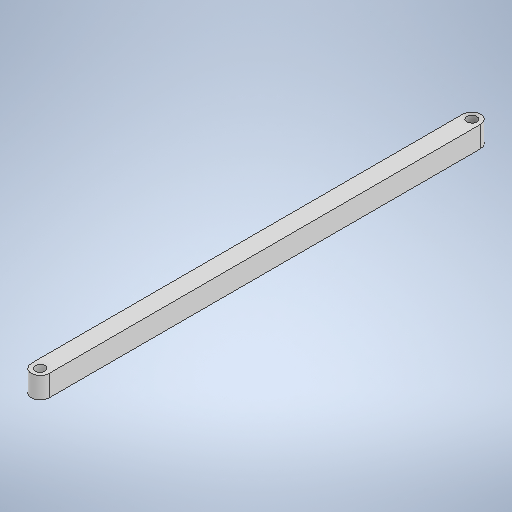
# Autodesk Inventor part: scrambler_spider_support1
Saved by Autodesk Inventor 2025.2 (Build 292293000, 293)
## iProperties
Created: 2025-10-14
Part Number: scrambler_spider_support1
Material: Generic
Document SubType Name: Modeling
Designer: pascu
Density: 1 g/cm^3
Appearance: Default
Author: pascu
Autodesk Inventor part; units mm, degrees
ref_plane "YZ Plane" through (0, 0, 0) normal (1, 0, 0) x (0, 1, 0)
ref_plane "XZ Plane" through (0, 0, 0) normal (0, 1, 0) x (-1, 0, 0)
ref_plane "XY Plane" through (0, 0, 0) normal (0, 0, 1) x (1, 0, 0)
sketch "Sketch1" plane through (0, 0, 0) normal (0, 1, 0) x (-1, 0, 0)
  line L0 (0, 0) -> (-3.175, 0)
  line L1 (-3.175, 0) -> (-3.175, -80.7212)
  line L2 (-3.175, -80.7212) -> (0, -80.7212)
  line L3 (0, -80.7212) -> (0, 0)
  dimension "d0" = 3.175
  dimension "d1" = 80.7212
  constraints: 8 end point, 2 parallel, 1 horizontal, 1 perpendicular
  measures "d0" distance of L2.end L1.end
  measures "d1" distance of L1.end L0.end
extrude "Extrusion1" add sketch "Sketch1" along normal blind 3.81
fillet "Fillet1" radius 1.5875 4 edges at (3.175, 1.905, 0) (0, 1.905, 0) (3.175, 1.905, -80.7212) (0, 1.905, -80.7212)
sketch "Sketch2" plane through (0, 3.81, 0) normal (0, 1, 0) x (1, 0, 0)
  arc A0 (0, 1.5875) -> (3.175, 1.5875) centre (1.5875, 1.5875) ccw projected
  circle A1 centre (1.5875, 1.5875) radius 0.889
  arc A2 (3.175, 79.1337) -> (0, 79.1337) centre (1.5875, 79.1337) ccw projected
  circle A3 centre (1.5875, 79.1337) radius 0.889
  point P0 (0, 0)
  dimension "d5" = 1.778
  dimension "d6" = 1.778
  constraints: 2 centre point, 2 coincident
  measures "d5" diameter of A1
  measures "d6" diameter of A3
extrude "Extrusion2" cut sketch "Sketch2" against normal blind 3.81
body "Solid1"
